Autodesk Fusion 360 part; units mm, degrees
(part 3 of 3)
  spline S53 degree 3 poles (-72.7696, -95.6386) (-72.7696, -96.5164) (-72.058, -97.228) (-71.1802, -97.228) knots 0 0 0 0 1 1 1 1
  line L259 (-71.1802, -97.228) -> (-69.6399, -97.228)
  spline S54 degree 3 poles (-69.6399, -97.228) (-68.7621, -97.228) (-67.3044, -97.2) (-66.5048, -97.547) knots 0 0 0 0 1 1 1 1
  spline S55 degree 3 poles (-66.5048, -97.547) (-65.6086, -97.936) (-64.8906, -98.654) (-64.5016, -99.5503) knots 0 0 0 0 1 1 1 1
  spline S56 degree 3 poles (-64.5016, -99.5503) (-64.1545, -100.3498) (-64.1826, -101.8075) (-64.1826, -102.6853) knots 0 0 0 0 1 1 1 1
  line L260 (-64.1826, -102.6853) -> (-64.1826, -112.1193)
  spline S57 degree 3 poles (-64.1826, -112.1193) (-64.1826, -112.9971) (-63.471, -113.7087) (-62.5932, -113.7087) knots 0 0 0 0 1 1 1 1
  line L261 (-62.5932, -113.7087) -> (6.5285, -113.7087)
  line L262 (6.5285, -113.7087) -> (29.9385, -113.7087)
  line L263 (29.9385, -113.7087) -> (62.5801, -113.7087)
  spline S58 degree 3 poles (62.5801, -113.7087) (63.4579, -113.7087) (64.1695, -112.9971) (64.1695, -112.1193) knots 0 0 0 0 1 1 1 1
  line L264 (64.1695, -112.1193) -> (64.1695, -102.6853)
  spline S59 degree 3 poles (64.1695, -102.6853) (64.1695, -101.8075) (64.1414, -100.3498) (64.4885, -99.5503) knots 0 0 0 0 1 1 1 1
  spline S60 degree 3 poles (64.4885, -99.5503) (64.8776, -98.654) (65.5955, -97.936) (66.4918, -97.547) knots 0 0 0 0 1 1 1 1
  spline S61 degree 3 poles (66.4918, -97.547) (67.2913, -97.1999) (68.7491, -97.228) (69.6269, -97.228) knots 0 0 0 0 1 1 1 1
  line L265 (69.6269, -97.228) -> (71.1671, -97.228)
  spline S62 degree 3 poles (71.1671, -97.228) (72.0449, -97.228) (72.7565, -96.5164) (72.7565, -95.6386) knots 0 0 0 0 1 1 1 1
  line L266 (72.7565, -95.6386) -> (72.7565, -78.342)
  line L267 (72.7565, -78.342) -> (72.7565, -69.9133)
  line L268 (72.7565, -69.9133) -> (72.7565, -30.6466)
  spline S63 degree 3 poles (72.7565, -30.6466) (72.7565, -29.7688) (72.0449, -29.0572) (71.1671, -29.0572) knots 0 0 0 0 1 1 1 1
  line L269 (71.1671, -29.0572) -> (69.9088, -29.0572)
  spline S64 degree 3 poles (69.9088, -29.0572) (69.031, -29.0572) (67.5733, -29.0853) (66.7737, -28.7382) knots 0 0 0 0 1 1 1 1
  spline S65 degree 3 poles (66.7737, -28.7382) (65.8776, -28.3492) (65.1599, -27.6312) (64.7709, -26.735) knots 0 0 0 0 1 1 1 1
  spline S66 degree 3 poles (64.7709, -26.735) (64.4239, -25.9354) (64.452, -24.4777) (64.452, -23.5999) knots 0 0 0 0 1 1 1 1
  line L270 (64.452, -23.5999) -> (64.452, -6.9154)
  spline S67 degree 3 poles (64.452, -6.9154) (64.452, -6.0376) (64.4239, -4.5799) (64.7709, -3.7803) knots 0 0 0 0 1 1 1 1
  spline S68 degree 3 poles (64.7709, -3.7803) (65.1599, -2.884) (65.8776, -2.1661) (66.7737, -1.7771) knots 0 0 0 0 1 1 1 1
  spline S69 degree 3 poles (66.7737, -1.7771) (67.5733, -1.4299) (69.031, -1.458) (69.9088, -1.458) knots 0 0 0 0 1 1 1 1
  line L271 (69.9088, -1.458) -> (71.1671, -1.458)
  spline S70 degree 3 poles (71.1671, -1.458) (72.0449, -1.458) (72.7565, -0.7464) (72.7565, 0.1314) knots 0 0 0 0 1 1 1 1
  line L272 (72.7565, 0.1314) -> (72.7565, 90.8652)
  spline S71 degree 3 poles (72.7565, 90.8652) (72.7565, 91.743) (72.0449, 92.4546) (71.1671, 92.4546) knots 0 0 0 0 1 1 1 1
  line L273 (71.1671, 92.4546) -> (69.9088, 92.4546)
  spline S72 degree 3 poles (69.9088, 92.4546) (69.031, 92.4546) (67.5733, 92.4265) (66.7737, 92.7736) knots 0 0 0 0 1 1 1 1
  spline S73 degree 3 poles (66.7737, 92.7736) (65.8776, 93.1626) (65.1599, 93.8805) (64.7709, 94.7768) knots 0 0 0 0 1 1 1 1
  spline S74 degree 3 poles (64.7709, 94.7768) (64.4239, 95.5764) (64.452, 97.0341) (64.452, 97.9119) knots 0 0 0 0 1 1 1 1
  spline S75 degree 3 poles (64.452, 97.9119) (64.452, 98.5551) (64.4239, 99.8226) (64.7709, 100.6222) knots 0 0 0 0 1 1 1 1
  spline S76 degree 3 poles (64.7709, 100.6222) (65.1599, 101.5185) (65.8776, 102.2364) (66.7737, 102.6254) knots 0 0 0 0 1 1 1 1
  spline S77 degree 3 poles (66.7737, 102.6254) (67.5733, 102.9726) (69.031, 102.9445) (69.9088, 102.9445) knots 0 0 0 0 1 1 1 1
  line L274 (69.9088, 102.9445) -> (71.1671, 102.9445)
  spline S78 degree 3 poles (71.1671, 102.9445) (72.0449, 102.9445) (72.7565, 103.6561) (72.7565, 104.5339) knots 0 0 0 0 1 1 1 1
  line L275 (72.7565, 104.5339) -> (72.7565, 111.3196)
  spline S79 degree 3 poles (72.7565, 111.3196) (72.7565, 111.3349) (72.7565, 111.3596) (72.7563, 111.3749) knots 0 0 0 0 1 1 1 1
  line L276 (57.9278, 7.8225) -> (57.9278, 1.8208)
  arc A257 (57.9278, 1.8208) -> (56.8913, 0.7844) centre (56.8913, 1.8208) cw
  line L277 (56.8913, 0.7844) -> (51.2209, 0.7844)
  arc A258 (51.2209, 0.7844) -> (50.1844, 1.8208) centre (51.2209, 1.8208) cw
  line L278 (50.1844, 1.8208) -> (50.1844, 7.8225)
  arc A259 (50.1844, 7.8225) -> (51.2209, 8.859) centre (51.2209, 7.8225) cw
  line L279 (51.2209, 8.859) -> (56.8913, 8.859)
  arc A260 (56.8913, 8.859) -> (57.9278, 7.8225) centre (56.8913, 7.8225) cw
  line L280 (57.9278, -5.0055) -> (57.9278, -11.0072)
  arc A261 (57.9278, -11.0072) -> (56.8913, -12.0436) centre (56.8913, -11.0072) cw
  line L281 (56.8913, -12.0436) -> (51.2209, -12.0436)
  arc A262 (51.2209, -12.0436) -> (50.1844, -11.0072) centre (51.2209, -11.0072) cw
  line L282 (50.1844, -11.0072) -> (50.1844, -5.0055)
  arc A263 (50.1844, -5.0055) -> (51.2209, -3.969) centre (51.2209, -5.0055) cw
  line L283 (51.2209, -3.969) -> (56.8913, -3.969)
  arc A264 (56.8913, -3.969) -> (57.9278, -5.0055) centre (56.8913, -5.0055) cw
  line L284 (31.3942, -79.7335) -> (39.4061, -79.7335)
  line L285 (40.4061, -80.7335) -> (40.4061, -88.7454)
  line L286 (39.4061, -89.7454) -> (31.3942, -89.7454)
  line L287 (30.3942, -88.7454) -> (30.3942, -80.7335)
  arc A265 (31.3942, -79.7335) -> (30.3942, -80.7335) centre (31.3942, -80.7335) ccw
  arc A266 (40.4061, -80.7335) -> (39.4061, -79.7335) centre (39.4061, -80.7335) ccw
  arc A267 (39.4061, -89.7454) -> (40.4061, -88.7454) centre (39.4061, -88.7454) ccw
  arc A268 (30.3942, -88.7454) -> (31.3942, -89.7454) centre (31.3942, -88.7454) ccw
  line L288 (16.2642, -79.7335) -> (24.2761, -79.7335)
  line L289 (25.2761, -80.7335) -> (25.2761, -88.7454)
  line L290 (24.2761, -89.7454) -> (16.2642, -89.7454)
  line L291 (15.2642, -88.7454) -> (15.2642, -80.7335)
  line L292 (1.0995, -79.7335) -> (9.1114, -79.7335)
  line L293 (10.1114, -80.7335) -> (10.1114, -88.7454)
  line L294 (9.1114, -89.7454) -> (1.0995, -89.7454)
  line L295 (0.0995, -88.7454) -> (0.0995, -80.7335)
  line L296 (-13.9253, -79.7335) -> (-5.9134, -79.7335)
  line L297 (-4.9134, -80.7335) -> (-4.9134, -88.7454)
  line L298 (-5.9134, -89.7454) -> (-13.9253, -89.7454)
  line L299 (-14.9253, -88.7454) -> (-14.9253, -80.7335)
  arc A269 (25.2761, -80.7335) -> (24.2761, -79.7335) centre (24.2761, -80.7335) ccw
  arc A270 (24.2761, -89.7454) -> (25.2761, -88.7454) centre (24.2761, -88.7454) ccw
  arc A271 (15.2642, -88.7454) -> (16.2642, -89.7454) centre (16.2642, -88.7454) ccw
  arc A272 (16.2642, -79.7335) -> (15.2642, -80.7335) centre (16.2642, -80.7335) ccw
  arc A273 (10.1114, -80.7335) -> (9.1114, -79.7335) centre (9.1114, -80.7335) ccw
  arc A274 (9.1114, -89.7454) -> (10.1114, -88.7454) centre (9.1114, -88.7454) ccw
  arc A275 (0.0995, -88.7454) -> (1.0995, -89.7454) centre (1.0995, -88.7454) ccw
  arc A276 (1.0995, -79.7335) -> (0.0995, -80.7335) centre (1.0995, -80.7335) ccw
  arc A277 (-4.9134, -80.7335) -> (-5.9134, -79.7335) centre (-5.9134, -80.7335) ccw
  arc A278 (-5.9134, -89.7454) -> (-4.9134, -88.7454) centre (-5.9134, -88.7454) ccw
  arc A279 (-14.9253, -88.7454) -> (-13.9253, -89.7454) centre (-13.9253, -88.7454) ccw
  arc A280 (-13.9253, -79.7335) -> (-14.9253, -80.7335) centre (-13.9253, -80.7335) ccw
  point P0 (69.6074, 107.2798)
  point P1 (-66.7683, 107.225)
  point P2 (69.6217, 2.396)
  point P3 (-66.8039, 2.3679)
  point P4 (69.5851, -93.0365)
  point P5 (-66.8388, -93)
  dimension "d12" = 1
  dimension "d13" = 1
  constraint horizontal L284
  constraint vertical L285
  constraint horizontal L286
  constraint vertical L287
  constraint tangent L284 A265
  constraint tangent L287 A265
  constraint tangent L284 A266
  constraint tangent L285 A266
  constraint equal A265 A266
  constraint tangent L285 A267
  constraint tangent L286 A267
  constraint equal A265 A267
  constraint tangent L286 A268
  constraint tangent L287 A268
  constraint equal A265 A268
  constraint horizontal L288
  constraint vertical L289
  constraint horizontal L290
  constraint vertical L291
  constraint horizontal L292
  constraint vertical L293
  constraint horizontal L294
  constraint vertical L295
  constraint horizontal L296
  constraint vertical L297
  constraint horizontal L298
  constraint vertical L299
  constraint tangent L288 A269
  constraint tangent L289 A269
  constraint tangent L289 A270
  constraint tangent L290 A270
  constraint equal A269 A270
  constraint tangent L290 A271
  constraint tangent L291 A271
  constraint equal A269 A271
  constraint tangent L288 A272
  constraint tangent L291 A272
  constraint equal A269 A272
  constraint tangent L292 A273
  constraint tangent L293 A273
  constraint equal A269 A273
  constraint tangent L293 A274
  constraint tangent L294 A274
  constraint equal A269 A274
  constraint tangent L294 A275
  constraint tangent L295 A275
  constraint equal A269 A275
  constraint tangent L292 A276
  constraint tangent L295 A276
  constraint equal A269 A276
  constraint tangent L296 A277
  constraint tangent L297 A277
  constraint equal A269 A277
  constraint tangent L297 A278
  constraint tangent L298 A278
  constraint equal A269 A278
  constraint tangent L298 A279
  constraint tangent L299 A279
  constraint equal A269 A279
  constraint tangent L296 A280
  constraint tangent L299 A280
  constraint equal A269 A280
  measures "d12" radius of A265
  measures "d13" radius of A269
extrude "Extrude2" add sketch "Middle" along normal blind 3
ref_plane "WorkPlane2" through (94.9965, -147.8775, 6) normal (0, 0, 1) x (1, 0, 0)
sketch "Sketch3" plane through (94.9965, -147.8775, 6) normal (0, 0, 1) x (1, 0, 0)
  spline S0 degree 3 poles (49.6233, 11.0815) (49.6233, 12.3941) (48.5663, 13.4506) (47.2536, 13.4506) knots 0 0 0 0 1 1 1 1
  line L0 (47.2536, 13.4506) -> (-22.1619, 13.4506)
  line L1 (-22.1619, 13.4506) -> (-48.9085, 13.4506)
  line L2 (-48.9085, 13.4506) -> (-56.7757, 13.4506)
  spline S1 degree 3 poles (-56.7757, 13.4506) (-58.0884, 13.4506) (-59.1448, 12.3941) (-59.1448, 11.0815) knots 0 0 0 0 1 1 1 1
  line L3 (-59.1448, 11.0815) -> (-59.1448, -51.7753)
  spline S2 degree 3 poles (-59.1448, -51.7753) (-59.1448, -53.088) (-58.0884, -54.1444) (-56.7757, -54.1444) knots 0 0 0 0 1 1 1 1
  line L4 (-56.7757, -54.1444) -> (-23.2215, -54.1444)
  spline S3 degree 3 poles (-23.2215, -54.1444) (-21.9089, -54.1444) (-20.8524, -53.088) (-20.8524, -51.7753) knots 0 0 0 0 1 1 1 1
  line L5 (-20.8524, -51.7753) -> (-20.8524, -16.8471)
  spline S4 degree 3 poles (-20.8524, -16.8471) (-20.8855, -15.835) (-20.1683, -15.2078) (-19.0718, -15.2078) knots 0 0 0 0 1 1 1 1
  line L6 (-19.0718, -15.2078) -> (47.2536, -15.2078)
  spline S5 degree 3 poles (47.2536, -15.2078) (48.5663, -15.2078) (49.6232, -14.1514) (49.6232, -12.8387) knots 0 0 0 0 1 1 1 1
  line L7 (49.6232, -12.8387) -> (49.6233, 11.0815)
  arc A0 (-54.8586, 0.849) -> (-55.8598, 1.8501) centre (-54.8586, 1.8501) cw
  line L8 (-54.8586, 0.849) -> (-43.6251, 0.849)
  arc A1 (-42.624, 1.8501) -> (-43.6251, 0.849) centre (-43.6251, 1.8501) cw
  line L9 (-42.624, 1.8501) -> (-42.6239, 7.9574)
  arc A2 (-43.6251, 8.9586) -> (-42.6239, 7.9574) centre (-43.6251, 7.9574) cw
  line L10 (-43.6251, 8.9586) -> (-54.8586, 8.9586)
  arc A3 (-55.8597, 7.9574) -> (-54.8586, 8.9586) centre (-54.8586, 7.9574) cw
  line L11 (-55.8597, 7.9574) -> (-55.8598, 1.8501)
  arc A4 (-54.8586, -11.968) -> (-55.8598, -10.9668) centre (-54.8586, -10.9668) cw
  line L12 (-54.8586, -11.968) -> (-43.6251, -11.968)
  arc A5 (-42.624, -10.9668) -> (-43.6251, -11.968) centre (-43.6251, -10.9668) cw
  line L13 (-42.624, -10.9668) -> (-42.6239, -4.8595)
  arc A6 (-43.6251, -3.8583) -> (-42.6239, -4.8595) centre (-43.6251, -4.8595) cw
  line L14 (-43.6251, -3.8583) -> (-54.8586, -3.8583)
  arc A7 (-55.8597, -4.8595) -> (-54.8586, -3.8583) centre (-54.8586, -4.8595) cw
  line L15 (-55.8597, -4.8595) -> (-55.8598, -10.9668)
  arc A8 (-36.9619, -11.968) -> (-37.9631, -10.9668) centre (-36.9619, -10.9668) cw
  line L16 (-36.9619, -11.968) -> (-25.7285, -11.968)
  arc A9 (-24.7273, -10.9668) -> (-25.7285, -11.968) centre (-25.7285, -10.9668) cw
  line L17 (-24.7273, -10.9668) -> (-24.7273, -4.8595)
  arc A10 (-25.7285, -3.8583) -> (-24.7273, -4.8595) centre (-25.7285, -4.8595) cw
  line L18 (-25.7285, -3.8583) -> (-36.9619, -3.8583)
  arc A11 (-37.9631, -4.8595) -> (-36.9619, -3.8583) centre (-36.9619, -4.8595) cw
  line L19 (-37.9631, -4.8595) -> (-37.9631, -10.9668)
  arc A12 (-36.9619, 0.849) -> (-37.9631, 1.8501) centre (-36.9619, 1.8501) cw
  line L20 (-36.9619, 0.849) -> (-25.7285, 0.849)
  arc A13 (-24.7273, 1.8501) -> (-25.7285, 0.849) centre (-25.7285, 1.8501) cw
  line L21 (-24.7273, 1.8501) -> (-24.7273, 7.9574)
  arc A14 (-25.7285, 8.9586) -> (-24.7273, 7.9574) centre (-25.7285, 7.9574) cw
  line L22 (-25.7285, 8.9586) -> (-36.9619, 8.9586)
  arc A15 (-37.9631, 7.9574) -> (-36.9619, 8.9586) centre (-36.9619, 7.9574) cw
  line L23 (-37.9631, 7.9574) -> (-37.9631, 1.8501)
  arc A16 (-18.8015, 0.849) -> (-19.8027, 1.8501) centre (-18.8015, 1.8501) cw
  line L24 (-18.8015, 0.849) -> (-7.5681, 0.849)
  arc A17 (-6.5669, 1.8501) -> (-7.5681, 0.849) centre (-7.5681, 1.8501) cw
  line L25 (-6.5669, 1.8501) -> (-6.5669, 7.9574)
  arc A18 (-7.5681, 8.9586) -> (-6.5669, 7.9574) centre (-7.5681, 7.9574) cw
  line L26 (-7.5681, 8.9586) -> (-18.8015, 8.9586)
  arc A19 (-19.8027, 7.9574) -> (-18.8015, 8.9586) centre (-18.8015, 7.9574) cw
  line L27 (-19.8027, 7.9574) -> (-19.8027, 1.8501)
  arc A20 (-18.8015, -11.968) -> (-19.8027, -10.9668) centre (-18.8015, -10.9668) cw
  line L28 (-18.8015, -11.968) -> (-7.5681, -11.968)
  arc A21 (-6.5669, -10.9668) -> (-7.5681, -11.968) centre (-7.5681, -10.9668) cw
  line L29 (-6.5669, -10.9668) -> (-6.5669, -4.8595)
  arc A22 (-7.5681, -3.8583) -> (-6.5669, -4.8595) centre (-7.5681, -4.8595) cw
  line L30 (-7.5681, -3.8583) -> (-18.8015, -3.8583)
  arc A23 (-19.8027, -4.8595) -> (-18.8015, -3.8583) centre (-18.8015, -4.8595) cw
  line L31 (-19.8027, -4.8595) -> (-19.8027, -10.9668)
  arc A24 (-0.6145, 0.849) -> (-1.6157, 1.8501) centre (-0.6145, 1.8501) cw
  line L32 (-0.6145, 0.849) -> (10.6189, 0.849)
  arc A25 (11.6201, 1.8501) -> (10.6189, 0.849) centre (10.6189, 1.8501) cw
  line L33 (11.6201, 1.8501) -> (11.6201, 7.9574)
  arc A26 (10.6189, 8.9586) -> (11.6201, 7.9574) centre (10.6189, 7.9574) cw
  line L34 (10.6189, 8.9586) -> (-0.6145, 8.9586)
  arc A27 (-1.6157, 7.9574) -> (-0.6145, 8.9586) centre (-0.6145, 7.9574) cw
  line L35 (-1.6157, 7.9574) -> (-1.6157, 1.8501)
  arc A28 (-0.6145, -11.968) -> (-1.6157, -10.9668) centre (-0.6145, -10.9668) cw
  line L36 (-0.6145, -11.968) -> (10.6189, -11.968)
  arc A29 (11.6201, -10.9668) -> (10.6189, -11.968) centre (10.6189, -10.9668) cw
  line L37 (11.6201, -10.9668) -> (11.6201, -4.8595)
  arc A30 (10.6189, -3.8583) -> (11.6201, -4.8595) centre (10.6189, -4.8595) cw
  line L38 (10.6189, -3.8583) -> (-0.6145, -3.8583)
  arc A31 (-1.6157, -4.8595) -> (-0.6145, -3.8583) centre (-0.6145, -4.8595) cw
  line L39 (-1.6157, -4.8595) -> (-1.6157, -10.9668)
  arc A32 (17.387, 0.849) -> (16.3858, 1.8501) centre (17.387, 1.8501) cw
  line L40 (17.387, 0.849) -> (28.6204, 0.849)
  arc A33 (29.6216, 1.8501) -> (28.6204, 0.849) centre (28.6204, 1.8501) cw
  line L41 (29.6216, 1.8501) -> (29.6216, 7.9574)
  arc A34 (28.6204, 8.9586) -> (29.6216, 7.9574) centre (28.6204, 7.9574) cw
  line L42 (28.6204, 8.9586) -> (17.387, 8.9586)
  arc A35 (16.3858, 7.9574) -> (17.387, 8.9586) centre (17.387, 7.9574) cw
  line L43 (16.3858, 7.9574) -> (16.3858, 1.8501)
  arc A36 (17.387, -11.968) -> (16.3858, -10.9668) centre (17.387, -10.9668) cw
  line L44 (17.387, -11.968) -> (28.6204, -11.968)
  arc A37 (29.6216, -10.9668) -> (28.6204, -11.968) centre (28.6204, -10.9668) cw
  line L45 (29.6216, -10.9668) -> (29.6216, -4.8595)
  arc A38 (28.6204, -3.8583) -> (29.6216, -4.8595) centre (28.6204, -4.8595) cw
  line L46 (28.6204, -3.8583) -> (17.387, -3.8583)
  arc A39 (16.3858, -4.8595) -> (17.387, -3.8583) centre (17.387, -4.8595) cw
  line L47 (16.3858, -4.8595) -> (16.3858, -10.9668)
  arc A40 (35.468, 0.849) -> (34.4668, 1.8501) centre (35.468, 1.8501) cw
  line L48 (35.468, 0.849) -> (46.7014, 0.849)
  arc A41 (47.7026, 1.8501) -> (46.7014, 0.849) centre (46.7014, 1.8501) cw
  line L49 (47.7026, 1.8501) -> (47.7026, 7.9574)
  arc A42 (46.7014, 8.9586) -> (47.7026, 7.9574) centre (46.7014, 7.9574) cw
  line L50 (46.7014, 8.9586) -> (35.468, 8.9586)
  arc A43 (34.4668, 7.9574) -> (35.468, 8.9586) centre (35.468, 7.9574) cw
  line L51 (34.4668, 7.9574) -> (34.4668, 1.8501)
  arc A44 (35.468, -11.968) -> (34.4668, -10.9668) centre (35.468, -10.9668) cw
  line L52 (35.468, -11.968) -> (46.7014, -11.968)
  arc A45 (47.7026, -10.9668) -> (46.7014, -11.968) centre (46.7014, -10.9668) cw
  line L53 (47.7026, -10.9668) -> (47.7026, -4.8595)
  arc A46 (46.7014, -3.8583) -> (47.7026, -4.8595) centre (46.7014, -4.8595) cw
  line L54 (46.7014, -3.8583) -> (35.468, -3.8583)
  arc A47 (34.4668, -4.8595) -> (35.468, -3.8583) centre (35.468, -4.8595) cw
  line L55 (34.4668, -4.8595) -> (34.4668, -10.9668)
  arc A48 (-54.8586, -25.3676) -> (-55.8598, -24.3664) centre (-54.8586, -24.3664) cw
  line L56 (-54.8586, -25.3676) -> (-43.6251, -25.3676)
  arc A49 (-42.624, -24.3664) -> (-43.6251, -25.3676) centre (-43.6251, -24.3664) cw
  line L57 (-42.624, -24.3664) -> (-42.6239, -18.2591)
  arc A50 (-43.6251, -17.2579) -> (-42.6239, -18.2591) centre (-43.6251, -18.2591) cw
  line L58 (-43.6251, -17.2579) -> (-54.8586, -17.2579)
  arc A51 (-55.8597, -18.2591) -> (-54.8586, -17.2579) centre (-54.8586, -18.2591) cw
  line L59 (-55.8597, -18.2591) -> (-55.8598, -24.3664)
  arc A52 (-54.8586, -38.4554) -> (-55.8598, -37.4542) centre (-54.8586, -37.4542) cw
  line L60 (-54.8586, -38.4554) -> (-43.6251, -38.4554)
  arc A53 (-42.624, -37.4542) -> (-43.6251, -38.4554) centre (-43.6251, -37.4542) cw
  line L61 (-42.624, -37.4542) -> (-42.6239, -31.347)
  arc A54 (-43.6251, -30.3458) -> (-42.6239, -31.347) centre (-43.6251, -31.347) cw
  line L62 (-43.6251, -30.3458) -> (-54.8586, -30.3458)
  arc A55 (-55.8597, -31.347) -> (-54.8586, -30.3458) centre (-54.8586, -31.347) cw
  line L63 (-55.8597, -31.347) -> (-55.8598, -37.4542)
  arc A56 (-54.8586, -51.4902) -> (-55.8598, -50.489) centre (-54.8586, -50.489) cw
  line L64 (-54.8586, -51.4902) -> (-43.6251, -51.4902)
  arc A57 (-42.624, -50.489) -> (-43.6251, -51.4902) centre (-43.6251, -50.489) cw
  line L65 (-42.624, -50.489) -> (-42.6239, -44.3817)
  arc A58 (-43.6251, -43.3805) -> (-42.6239, -44.3817) centre (-43.6251, -44.3817) cw
  line L66 (-43.6251, -43.3805) -> (-54.8586, -43.3805)
  arc A59 (-55.8597, -44.3817) -> (-54.8586, -43.3805) centre (-54.8586, -44.3817) cw
  line L67 (-55.8597, -44.3817) -> (-55.8598, -50.489)
  arc A60 (-36.9619, -51.4902) -> (-37.9631, -50.489) centre (-36.9619, -50.489) cw
  line L68 (-36.9619, -51.4902) -> (-25.7285, -51.4902)
  arc A61 (-24.7273, -50.489) -> (-25.7285, -51.4902) centre (-25.7285, -50.489) cw
  line L69 (-24.7273, -50.489) -> (-24.7273, -44.3817)
  arc A62 (-25.7285, -43.3805) -> (-24.7273, -44.3817) centre (-25.7285, -44.3817) cw
  line L70 (-25.7285, -43.3805) -> (-36.9619, -43.3805)
  arc A63 (-37.9631, -44.3817) -> (-36.9619, -43.3805) centre (-36.9619, -44.3817) cw
  line L71 (-37.9631, -44.3817) -> (-37.9631, -50.489)
  arc A64 (-36.9619, -38.4554) -> (-37.9631, -37.4542) centre (-36.9619, -37.4542) cw
  line L72 (-36.9619, -38.4554) -> (-25.7285, -38.4554)
  arc A65 (-24.7273, -37.4542) -> (-25.7285, -38.4554) centre (-25.7285, -37.4542) cw
  line L73 (-24.7273, -37.4542) -> (-24.7273, -31.347)
  arc A66 (-25.7285, -30.3458) -> (-24.7273, -31.347) centre (-25.7285, -31.347) cw
  line L74 (-25.7285, -30.3458) -> (-36.9619, -30.3458)
  arc A67 (-37.9631, -31.347) -> (-36.9619, -30.3458) centre (-36.9619, -31.347) cw
  line L75 (-37.9631, -31.347) -> (-37.9631, -37.4542)
  arc A68 (-36.9619, -25.3676) -> (-37.9631, -24.3664) centre (-36.9619, -24.3664) cw
  line L76 (-36.9619, -25.3676) -> (-25.7285, -25.3676)
  arc A69 (-24.7273, -24.3664) -> (-25.7285, -25.3676) centre (-25.7285, -24.3664) cw
  line L77 (-24.7273, -24.3664) -> (-24.7273, -18.2591)
  arc A70 (-25.7285, -17.2579) -> (-24.7273, -18.2591) centre (-25.7285, -18.2591) cw
  line L78 (-25.7285, -17.2579) -> (-36.9619, -17.2579)
  arc A71 (-37.9631, -18.2591) -> (-36.9619, -17.2579) centre (-36.9619, -18.2591) cw
  line L79 (-37.9631, -18.2591) -> (-37.9631, -24.3664)
extrude "Extrude3" add sketch "Sketch3" along normal blind 3
equation "layer_t = 3 mm" comment "Layer thickness"
equation "d4 = layer_t"
equation "d7 = layer_t"
equation "d10 = layer_t"
